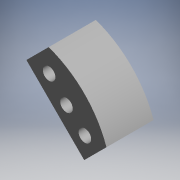
# Autodesk Inventor part: encoder_sensor
Saved by Autodesk Inventor 2019.4 (Build 234330000, 330)
## iProperties
Created: 2020-06-20
Part Number: encoder_sensor
Material: Generic
Document SubType Name: Modeling
Designer: Jorge
Density: 1 g/cm^3
Appearance: Default
Author: Jorge
Autodesk Inventor part; units mm, degrees
ref_plane "YZ Plane" through (0, 0, 0) normal (1, 0, 0) x (0, 1, 0)
ref_plane "XZ Plane" through (0, 0, 0) normal (0, 1, 0) x (-1, 0, 0)
ref_plane "XY Plane" through (0, 0, 0) normal (0, 0, 1) x (1, 0, 0)
sketch "Sketch1" plane through (0, 0, 0) normal (0, 0, 1) x (1, 0, 0)
  circle A0 centre (0, 0) radius 0.5 projected
  circle A1 centre (1.4639, -1.3645) radius 0.5 projected
  circle A2 centre (-1.3812, 1.4806) radius 0.5 projected
  circle A3 centre (4.5267, -2.6595) radius 0.5 projected
  circle A4 centre (6.5905, -2.6595) radius 0.5 projected
  circle A5 centre (8.6472, -2.6595) radius 0.5 projected
  line L0 (1.4639, -1.3645) -> (-1.3812, 1.4806) construction
  line L1 (-3.1847, 1.5164) -> (1.4115, -3.0798)
  line L2 (1.4115, -3.0798) -> (3.1792, -1.312)
  line L3 (3.1792, -1.312) -> (-1.417, 3.2842) construction
  line L4 (-1.417, 3.2842) -> (-3.1847, 1.5164)
  arc A6 (3.1792, -1.312) -> (-1.417, 3.2842) centre (-3.8329, -3.728) ccw
  point P0 (0, 0)
  dimension "d0" = 2.5
  dimension "d1" = 6.5
  constraints: 10 end point, 3 perpendicular, 2 point on circle, 1 centre point, 1 other
  measures "d0" distance of L3.end L1.start
  measures "d1" distance of L2.end L3.end
extrude "Extrusion1" add sketch "Sketch1" along normal blind 3.75 contours L4 A6 L2 L1
body "Solid1"
